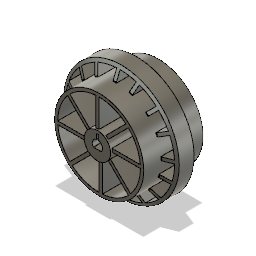
_k346 improved hub- tuned for my ender3.f68e6394-e35d-43b5-a4ef-b5a22b10e9ee (Autodesk Fusion 360 design; units mm, degrees)
Autodesk Fusion 360 part; units mm, degrees
sketch "Sketch1" plane through (0, 0, 0) normal (0, 0, 1) x (1, 0, 0)
  circle A0 centre (0, 0) radius 17.5
  line L0 (-2.8284, 2.8284) -> (-8.8388, 8.8388)
  line L1 (-2.8284, -2.8284) -> (-8.8388, -8.8388)
  line L2 (2.8284, -2.8284) -> (8.8388, -8.8388)
  line L3 (4, 0) -> (12.5, 0)
  line L4 (-4, 0) -> (-12.5, 0)
  line L5 (0, -4) -> (0, -12.5)
  line L6 (4, 0) -> (13.5, 0) construction
  line L7 (2.8284, 2.8284) -> (8.8388, 8.8388)
  line L8 (0, 4) -> (0, 12.5)
  arc A1 (9.5459, 9.5459) -> (13.4629, 1) centre (0, 0) ccw
  line L9 (4, 0) -> (12.5, 0) construction
  line L10 (-12.5, 0) -> (-4, 0)
  arc A2 (-3.4457, 2.0315) -> (-4, 0) centre (0, 0) ccw
  arc A3 (-1, 3.873) -> (-2.8284, 2.8284) centre (0, 0) ccw
  arc A4 (2.0315, 3.4457) -> (0, 4) centre (0, 0) ccw
  arc A5 (3.873, 1) -> (2.8284, 2.8284) centre (0, 0) ccw
  arc A6 (3.4457, -2.0315) -> (4, 0) centre (0, 0) ccw
  arc A7 (1, -3.873) -> (2.8284, -2.8284) centre (0, 0) ccw
  arc A8 (-3.873, -1) -> (-2.8284, -2.8284) centre (0, 0) ccw
  arc A9 (-2.0315, -3.4457) -> (0, -4) centre (0, 0) ccw
  arc A10 (-12.4599, -1) -> (-8.8388, -8.8388) centre (0, 0) ccw
  arc A11 (-8.1034, -9.5176) -> (0, -12.5) centre (0, 0) ccw
  arc A12 (1, -12.4599) -> (8.8388, -8.8388) centre (0, 0) ccw
  arc A13 (9.5176, -8.1034) -> (12.5, 0) centre (0, 0) ccw
  arc A14 (12.4599, 1) -> (8.8388, 8.8388) centre (0, 0) ccw
  arc A15 (8.1034, 9.5176) -> (0, 12.5) centre (0, 0) ccw
  arc A16 (-1, 12.4599) -> (-8.8388, 8.8388) centre (0, 0) ccw
  arc A17 (-9.5176, 8.1034) -> (-12.5, 0) centre (0, 0) ccw
  line L11 (-12.5, 0) -> (-4, 0)
  circle A18 centre (0, 0) radius 4
  line L12 (4.9142, 15.7829) -> (3.8375, 12.9431)
  line L13 (5.8492, 15.4284) -> (4.7857, 12.6233)
  line L14 (-7.6854, 14.6351) -> (-6.4386, 11.8657)
  line L15 (-6.7735, 15.0456) -> (-5.542, 12.31)
  line L16 (-15.4284, 5.8492) -> (-12.6233, 4.7857)
  line L17 (-15.7829, 4.9142) -> (-12.9431, 3.8375)
  line L18 (-15.0456, -6.7735) -> (-12.31, -5.542)
  line L19 (-14.6351, -7.6854) -> (-11.8657, -6.4386)
  line L20 (-5.8492, -15.4284) -> (-4.7857, -12.6233)
  line L21 (-4.9142, -15.7829) -> (-3.8375, -12.9431)
  line L22 (6.7735, -15.0456) -> (5.542, -12.31)
  line L23 (7.6854, -14.6351) -> (6.4386, -11.8657)
  line L24 (15.4284, -5.8492) -> (12.6233, -4.7857)
  line L25 (15.7829, -4.9142) -> (12.9431, -3.8375)
  line L26 (15.0456, 6.7735) -> (12.31, 5.542)
  line L27 (14.6351, 7.6854) -> (11.8657, 6.4386)
  arc A19 (16.4697, 1) -> (15.0456, 6.7735) centre (0, 0) ccw
  arc A20 (14.6074, 7.6729) -> (11.6673, 11.6673) centre (0, 0) ccw
  arc A21 (12.3529, -10.9387) -> (15.4284, -5.8492) centre (0, 0) ccw
  arc A22 (15.7546, -4.9034) -> (16.5, 0) centre (0, 0) ccw
  arc A23 (1, -16.4697) -> (6.7735, -15.0456) centre (0, 0) ccw
  arc A24 (7.6729, -14.6074) -> (11.6673, -11.6673) centre (0, 0) ccw
  arc A25 (-10.9387, -12.3529) -> (-5.8492, -15.4284) centre (0, 0) ccw
  arc A26 (-4.9034, -15.7546) -> (0, -16.5) centre (0, 0) ccw
  arc A27 (-16.4697, -1) -> (-15.0456, -6.7735) centre (0, 0) ccw
  arc A28 (-14.6074, -7.6729) -> (-11.6673, -11.6673) centre (0, 0) ccw
  arc A29 (-12.3529, 10.9387) -> (-15.4284, 5.8492) centre (0, 0) ccw
  arc A30 (-15.7546, 4.9034) -> (-16.5, 0) centre (0, 0) ccw
  arc A31 (-1, 16.4697) -> (-6.7735, 15.0456) centre (0, 0) ccw
  arc A32 (-7.6729, 14.6074) -> (-11.6673, 11.6673) centre (0, 0) ccw
  arc A33 (10.9387, 12.3529) -> (5.8492, 15.4284) centre (0, 0) ccw
  arc A34 (4.9034, 15.7546) -> (0, 16.5) centre (0, 0) ccw
  line L28 (-1.1843, -1) -> (1.1843, -1)
  line L29 (4, 0) -> (45, 0) construction
  line L30 (4, 0) -> (12.5, 0) construction
  line L31 (4, 0) -> (12.5, 0) construction
  line L32 (4, 0) -> (12.5, 0)
  line L33 (13.5, 0) -> (16.5, 0)
  line L34 (3.873, 1) -> (12.4599, 1)
  line L35 (13.4629, 1) -> (16.4697, 1)
  line L36 (11.6673, 11.6673) -> (9.5459, 9.5459)
  line L37 (8.8388, 8.8388) -> (2.8284, 2.8284)
  line L38 (10.9387, 12.3529) -> (8.8126, 10.2268)
  line L39 (8.1034, 9.5176) -> (2.0315, 3.4457)
  line L40 (0, 16.5) -> (0, 13.5)
  line L41 (0, 12.5) -> (0, 4)
  line L42 (-1, 16.4697) -> (-1, 13.4629)
  line L43 (-1, 12.4599) -> (-1, 3.873)
  line L44 (-11.6673, 11.6673) -> (-9.5459, 9.5459)
  line L45 (-8.8388, 8.8388) -> (-2.8284, 2.8284)
  line L46 (-12.3529, 10.9387) -> (-10.2268, 8.8126)
  line L47 (-9.5176, 8.1034) -> (-3.4457, 2.0315)
  line L48 (-16.4697, -1) -> (-13.4629, -1)
  line L49 (-12.4599, -1) -> (-3.873, -1)
  line L50 (-16.5, 0) -> (-13.5, 0)
  line L51 (-12.5, 0) -> (-4, 0)
  arc A35 (1, -13.4629) -> (12.9431, -3.8375) centre (0, 0) ccw
  line L52 (-11.6673, -11.6673) -> (-9.5459, -9.5459)
  line L53 (-8.8388, -8.8388) -> (-2.8284, -2.8284)
  arc A36 (13.4629, 1) -> (-11.8657, -6.4386) centre (0, 0) ccw
  arc A37 (-8.8126, -10.2268) -> (0, -13.5) centre (0, 0) ccw
  line L54 (-10.9387, -12.3529) -> (-8.8126, -10.2268)
  line L55 (-8.1034, -9.5176) -> (-2.0315, -3.4457)
  line L56 (0, -16.5) -> (0, -13.5)
  line L57 (0, -12.5) -> (0, -4)
  line L58 (1, -16.4697) -> (1, -13.4629)
  line L59 (1, -12.4599) -> (1, -3.873)
  line L60 (11.6673, -11.6673) -> (9.5459, -9.5459)
  line L61 (8.8388, -8.8388) -> (2.8284, -2.8284)
  line L62 (12.3529, -10.9387) -> (10.2268, -8.8126)
  line L63 (9.5176, -8.1034) -> (3.4457, -2.0315)
  line L64 (0.25, 1.5297) -> (0.25, 3)
  line L65 (-0.25, 1.5297) -> (-0.25, 3)
  line L66 (-0.25, 3) -> (0.25, 3)
  arc A38 (1.1843, -1) -> (0.25, 1.5297) centre (0, 0) ccw
  arc A39 (-0.25, 1.5297) -> (-1.1843, -1) centre (0, 0) ccw
  dimension "d1" = 35
  dimension "d5" = 8
  dimension "d6" = 3.1
  dimension "d20" = 13.5
  dimension "d22" = 25
  measures "d1" diameter of A0
  measures "d5" diameter of A8
  measures "d6" diameter of A38
  measures "d20" distance of A0.centre
  measures "d22" diameter of A10
extrude "Extrude2" add sketch "Sketch1" along normal blind 9 contours A2 A3 A4 A5 A6 A7 A8 A9 A18 | A1 A35 A36 A37 makes body 1
extrude "Extrude3" add sketch "Sketch1" along normal blind 3.75 contours A0 | L27 A20 L36 A36 | A1 L13 A33 L38 A36 | L26 A19 L35 A36 | A1 L12 A34 L40 A36 | A1 L25 A22 L33 | A1 L15 A31 L42 A36 | A1 L24 A21 A35 L62 | A1 L14 A32 L44 A36 | A1 L23 A24 A35 L60 | A1 L16 A29 L46 A36 | A1 L22 A23 A35 L58 | A1 L17 A30 L50 A36 | A1 L21 A26 A37 L56 | A1 L18 A27 L48 A36 | A1 L20 A25 A37 L54 | A1 L19 A28 L52 bodies 1
extrude "Extrude4" cut sketch "Sketch1" along normal blind 10 contours L27 A20 L36 A36 | A1 L13 A33 L38 A36 | L26 A19 L35 A36 | A1 L12 A34 L40 A36 | A1 L25 A22 L33 | A1 L15 A31 L42 A36 | A1 L24 A21 A35 L62 | A1 L14 A32 L44 A36 | A1 L23 A24 A35 L60 | A1 L16 A29 L46 A36 | A1 L22 A23 A35 L58 | A1 L17 A30 L50 A36 | A1 L21 A26 A37 L56 | A1 L18 A27 L48 A36 | A1 L20 A25 A37 L54 | A1 L19 A28 L52 bodies 1
extrude "Extrude5" add sketch "Sketch1" against normal blind 3.75 contours A0 bodies 1
extrude "Extrude6" add sketch "Sketch1" against normal blind 9 contours A2 A3 A4 A5 A6 A7 A8 A9 A18 | A1 A35 A36 A37 bodies 1
extrude "Extrude7" add sketch "Sketch1" along normal blind 9.5 contours A2 A3 A4 A5 A6 A7 A8 A9 A18 bodies 1
chamfer "Chamfer1" distance 3.75 distance2 1.5 2 edges at (-16.3157, 6.3283, -3.75) (-16.3157, -6.3283, 3.75) measured on face at (0, 17.134, -3.75) measured on face at (0, 17.134, 3.75) on bodies 1
extrude "Extrude8" add sketch "Sketch1" along normal blind 5 separate body contours A2 A3 A4 A5 A6 A7 A8 A9 A18 makes body 2
hidden bodies 2
